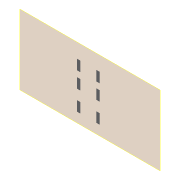
# Autodesk Inventor part: Stripes on the floor
Saved by Autodesk Inventor 2015 (Build 190159000, 159)
## iProperties
Created: 2015-04-12
Part Number: Stripes on the floor
Material: Generic
Document SubType Name: Modeling
Designer: Vukica
Density: 1 g/cm^3
Appearance: Default
Author: Vukica
Autodesk Inventor part; units mm, degrees
ref_plane "YZ Plane" through (0, 0, 0) normal (1, 0, 0) x (0, 1, 0)
ref_plane "XZ Plane" through (0, 0, 0) normal (0, 1, 0) x (-1, 0, 0)
ref_plane "XY Plane" through (0, 0, 0) normal (0, 0, 1) x (1, 0, 0)
ref_plane "Work Plane1" through (0, 0, 0) normal (0, 0, 1) x (1, 0, 0)
sketch "Sketch1" plane through (0, 0, 0) normal (0, 0, 1) x (1, 0, 0)
  line L0 (-368.3, 406.4) -> (-368.3, -406.4) projected
  line L1 (-368.3, 1092.2) -> (-368.3, 406.4) projected
  line L2 (241.3, 1092.2) -> (241.3, 406.4) projected
  line L3 (241.3, -406.4) -> (241.3, 406.4) projected
  line L4 (-368.3, -406.4) -> (-368.3, -1092.2) projected
  line L5 (241.3, -1092.2) -> (241.3, -406.4) projected
  line L6 (-368.3, 787.4) -> (-495.3, 787.4)
  line L7 (-495.3, 787.4) -> (-495.3, 406.4)
  line L8 (-495.3, 406.4) -> (-368.3, 406.4)
  line L9 (-368.3, 406.4) -> (-368.3, 787.4)
  line L10 (-368.3, 177.8) -> (-495.3, 177.8)
  line L11 (-495.3, 177.8) -> (-495.3, -203.2)
  line L12 (-495.3, -203.2) -> (-368.3, -203.2)
  line L13 (-368.3, -203.2) -> (-368.3, 177.8)
  line L14 (-368.3, -584.2) -> (-495.3, -584.2)
  line L15 (-495.3, -584.2) -> (-495.3, -965.2)
  line L16 (-495.3, -965.2) -> (-368.3, -965.2)
  line L17 (-368.3, -965.2) -> (-368.3, -584.2)
  line L18 (241.3, 787.4) -> (368.3, 787.4)
  line L19 (368.3, 787.4) -> (368.3, 406.4)
  line L20 (368.3, 406.4) -> (241.3, 406.4)
  line L21 (241.3, 406.4) -> (241.3, 787.4)
  line L22 (241.3, 177.8) -> (368.3, 177.8)
  line L23 (368.3, 177.8) -> (368.3, -203.2)
  line L24 (368.3, -203.2) -> (241.3, -203.2)
  line L25 (241.3, -203.2) -> (241.3, 177.8)
  line L26 (241.3, -584.2) -> (368.3, -584.2)
  line L27 (368.3, -584.2) -> (368.3, -965.2)
  line L28 (368.3, -965.2) -> (241.3, -965.2)
  line L29 (241.3, -965.2) -> (241.3, -584.2)
  line L30 (2438.4, 1219.2) -> (-2451.1, 1219.2) projected
  line L31 (-2451.1, -1219.2) -> (2438.4, -1219.2) projected
  point P0 (0, 0)
  dimension "d0" = 127
  dimension "d1" = 127
  dimension "d2" = 381
  dimension "d3" = 381
  dimension "d4" = 381
  dimension "d5" = 254
  dimension "d6" = 381
  dimension "d7" = 228.6
  constraints: 48 end point, 12 parallel, 9 point on line, 7 collinear, 6 horizontal, 6 perpendicular
  measures "d0" distance of L6.start L6.end
  measures "d1" distance of L18.start L18.end
  measures "d2" distance of L6.end L7.end
  measures "d3" distance of L10.end L11.end
  measures "d4" distance of L14.end L15.end
  measures "d5" distance between parallel lines of L31 L16
  measures "d6" distance between parallel lines of L12 L14
  measures "d7" distance between parallel lines of L8 L10
extrude "Extrusion1" add sketch "Sketch1" along normal blind 2.54
equation "\"d1\" = d0"
body "Solid1"
